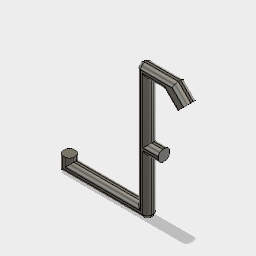
pegboard-hook-001 (Autodesk Fusion 360 design; units mm, degrees)
Autodesk Fusion 360 part; units mm, degrees
sketch "スケッチ3" plane through (0, 0, 0) normal (0, 1, 0) x (1, 0, 0)
  line L0 (5, -5) -> (10, -5)
  line L1 (10, -5) -> (10, -10)
  line L2 (10, -10) -> (5, -10)
  line L3 (5, -10) -> (5, -5)
  line L4 (-10, 0) -> (-5, 0)
  line L5 (-5, 0) -> (-5, 60)
  line L6 (-5, 60) -> (-10, 60)
  line L7 (-10, 60) -> (-10, 0)
  line L8 (10, 10) -> (10, 5)
  line L9 (10, 5) -> (17, 5)
  line L10 (17, 10) -> (10, 10)
  line L11 (-5, 55) -> (-10, 55)
  line L12 (-10, 55) -> (-10, 0)
  line L13 (-10, 0) -> (-5, 0)
  line L14 (-5, 0) -> (-5, 55)
  line L15 (5, 0) -> (10, 0)
  line L16 (10, 0) -> (10, 60)
  line L17 (10, 60) -> (5, 60)
  line L18 (5, 60) -> (5, 0)
  line L19 (-5, 10) -> (-5, 5)
  line L20 (-5, 5) -> (30, 5)
  line L21 (30, 5) -> (30, 10)
  line L22 (30, 10) -> (-5, 10)
  line L23 (17, 5) -> (17, 10)
  dimension "d4" = 5
  dimension "d5" = 5
  measures "d4" distance of L0 L2
  measures "d5" distance of L1 L3
  measures "d17" distance of L11.end
extrude "押し出し2" add sketch "スケッチ3" along normal blind 60 contours L0 L1 L2 L3
sketch "スケッチ4" plane through (10, 0, 0) normal (1, 0, 0) x (0, 0, -1)
  line L0 (-10, 0) -> (-5, 0)
  line L1 (-5, 0) -> (-5, 60)
  line L2 (-5, 60) -> (-10, 60)
  line L3 (-10, 60) -> (-10, 0)
  line L4 (-10, 60) -> (-5, 60)
  line L5 (-5, 60) -> (-5, 55)
  line L6 (-5, 55) -> (-10, 55)
  line L7 (-10, 55) -> (-10, 60)
  dimension "d10" = 5
  measures "d10" distance of L4 L6
extrude "押し出し4" add sketch "スケッチ4" along normal blind 12 contours L1 L2 L3 L4 L5 L6 L7
chamfer "面取り1" distance 5 angle 45 1 edges at (22, 55, 7.5)
extrude "押し出し9" add 1 faces at (20.3337, 58.3327, 6.6667) along direction (0.707107, -0.707107, 0) blind 8
sketch "スケッチ5" plane through (0, 55, 0) normal (0, -1, 0) x (1, 0, 0)
  line L0 (10, 10) -> (10, 5)
  line L1 (10, 5) -> (17, 5)
  line L2 (17, 10) -> (10, 10)
  line L3 (17, 10) -> (12, 10)
  line L4 (12, 10) -> (12, 5)
  line L5 (12, 5) -> (17, 5)
  line L6 (17, 5) -> (17, 10)
  line L7 (17, 5) -> (17, 10)
  dimension "d13" = 5
  measures "d13" distance of L4 L6
sketch "スケッチ7" plane through (10, 0, 0) normal (1, 0, 0) x (0, 0, -1)
  line L0 (-5, 55) -> (-10, 55)
  line L1 (-10, 55) -> (-10, 0)
  line L2 (-10, 0) -> (-5, 0)
  line L3 (-5, 0) -> (-5, 55)
  line L4 (-10, 30) -> (-5, 30)
  line L5 (-5, 30) -> (-5, 25)
  line L6 (-5, 25) -> (-10, 25)
  line L7 (-10, 25) -> (-10, 30)
  dimension "d17" = 25
  dimension "d18" = 5
  measures "d17" distance of L0.end L4
  measures "d18" distance of L4 L6
extrude "押し出し6" add sketch "スケッチ7" along normal blind 5 contours L1 L3 L4 L5 L6 L7
sketch "スケッチ8" plane through (5, 0, 0) normal (-1, 0, 0) x (0, 0, 1)
  line L0 (5, 0) -> (10, 0)
  line L1 (10, 0) -> (10, 60)
  line L2 (10, 60) -> (5, 60)
  line L3 (5, 60) -> (5, 0)
  line L4 (5, 0) -> (10, 0)
  line L5 (10, 0) -> (10, 5)
  line L6 (10, 5) -> (5, 5)
  line L7 (5, 5) -> (5, 0)
  dimension "d21" = 5
  measures "d21" distance of L4 L6
extrude "押し出し7" add sketch "スケッチ8" along normal blind 35 contours L0 L1 L3 L4 L5 L6 L7
sketch "スケッチ9" plane through (0, 5, 0) normal (0, 1, 0) x (-1, 0, 0)
  line L0 (-5, 10) -> (-5, 5)
  line L1 (-5, 5) -> (30, 5)
  line L2 (30, 5) -> (30, 10)
  line L3 (30, 10) -> (-5, 10)
  line L4 (30, 5) -> (25, 5)
  line L5 (25, 5) -> (25, 10)
  line L6 (25, 10) -> (30, 10)
  line L7 (30, 10) -> (30, 5)
  dimension "d24" = 5
  measures "d24" distance of L1.end L5
extrude "押し出し8" add sketch "スケッチ9" along normal blind 2 contours L1 L2 L3 L4 L5 L6 L7
fillet "フィレット6" radius 2 8 edges at (13.5, 60, 10) (13.5, 60, 5) (13.5, 55, 10) (13.5, 55, 5) (19.8284, 52.1716, 5) (24.8284, 57.1716, 5) (24.8284, 57.1716, 10) (19.8284, 52.1716, 10)
fillet "フィレット7" radius 2 13 edges at (5, 31.5, 5) (5, 59.4142, 5.5858) (5, 60, 7.5) (5, 59.4142, 9.4142) (5, 31.5, 10) (10, 43.5, 5) (10, 43.5, 10) (12.5, 30, 5) (12.5, 30, 10) (12.5, 25, 10) (10, 12.5, 10) (10, 12.5, 5) (12.5, 25, 5)
fillet "フィレット8" radius 2 11 edges at (-9, 5, 10) (-9, 5, 5) (-11, 0, 5) (9.4142, 0, 5.5858) (10, 0, 7.5) (9.4142, 0, 9.4142) (-11, 0, 10) (-30, 3.5, 5) (-30, 3.5, 10) (-25, 6, 10) (-25, 6, 5)
